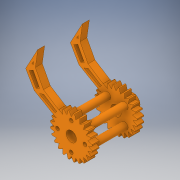
# Autodesk Inventor part: Relic arm front
Saved by Autodesk Inventor 2017 (Build 210142000, 142)
## iProperties
Created: 2018-01-06
Part Number: Relic arm front
Material: Generic
Document SubType Name: Modeling
Designer: Delta
Density: 1 g/cm^3
Appearance: Orange
Author: Delta
Autodesk Inventor part; units mm, degrees
ref_plane "YZ Plane" through (0, 0, 0) normal (1, 0, 0) x (0, 1, 0)
ref_plane "XZ Plane" through (0, 0, 0) normal (0, 1, 0) x (-1, 0, 0)
ref_plane "XY Plane" through (0, 0, 0) normal (0, 0, 1) x (1, 0, 0)
sketch "Sketch1" plane through (0, 0, 0) normal (0, 0, 1) x (1, 0, 0)
  line L0 (0, 0) -> (12.7, 0)
  line L1 (0, 0) -> (12.2673, 3.287)
  line L2 (0, 0) -> (12.7, 0) construction
  line L3 (12.2673, 3.287) -> (19.9534, 1.2275)
  line L4 (12.7, 0) -> (16.4514, 2.1659)
  line L5 (12.7, 0) -> (17.0317, 0) construction
  line L6 (16.4514, 2.1659) -> (12.7, 0)
  line L7 (16.4514, 2.1659) -> (12.2673, 3.287)
  line L8 (0, 0) -> (12.2673, 3.287)
  line L9 (16.4514, 2.1659) -> (12.7, 0)
  line L10 (0, 0) -> (12.7, 0)
  dimension "d0" = 12.7
  dimension "d1" = 12.7
  dimension "d2" = 15
  dimension "d3" = 150
  dimension "d4" = 30
  constraints: 22 end point, 3 horizontal, 2 collinear, 2 equal length, 1 point on line
  measures "d0" distance of L0.start L0.end
  measures "d1" distance of L0.start L1.end
  measures "d2" angle of L2 L1
  measures "d3" angle of L1 L3
  measures "d4" angle of L5 L4
extrude "Extrusion1" add sketch "Sketch1" along normal blind 5.08
sketch "Sketch2" plane through (0, 0, 5.08) normal (0, 0, 1) x (1, 0, 0)
  line L0 (0, 0) -> (12.7, 0) projected
  line L1 (16.4514, 2.1659) -> (12.2673, 3.287) projected
  line L2 (0, 0) -> (12.2673, 3.287)
  line L3 (0, 0) -> (10.9985, 6.35)
  line L4 (0, 0) -> (12.7, 0) construction
  line L5 (12.2673, 3.287) -> (13.7055, 5.7781)
  line L6 (12.2673, 3.287) -> (15.1438, 3.287) construction
  line L7 (13.7055, 5.7781) -> (10.829, 5.7781)
  line L8 (10.9985, 6.35) -> (14.0357, 6.35)
  line L9 (14.0357, 6.35) -> (13.7055, 5.7781)
  line L10 (12.2673, 3.287) -> (15.3303, 6.35)
  line L11 (15.3303, 6.35) -> (14.0357, 6.35)
  line L12 (12.2673, 3.287) -> (15.3303, 6.35)
  line L13 (10.9985, 6.35) -> (15.3303, 6.35)
  dimension "d7" = 12.7
  dimension "d8" = 30
  dimension "d9" = 60
  dimension "d10" = 60
  constraints: 24 end point, 3 horizontal, 2 collinear, 2 equal length, 1 point on line
  measures "d7" distance of L0.start L3.end
  measures "d8" angle of L4 L3
  measures "d9" angle of L6 L5
  measures "d10" angle of L7 L5
extrude "Extrusion2" add sketch "Sketch2" against normal blind 5.08
sketch "Sketch3" plane through (0, 0, 5.08) normal (0, 0, 1) x (1, 0, 0)
  line L0 (0, 0) -> (10.9985, 6.35) projected
  line L1 (0, 0) -> (10.9985, 6.35)
  line L2 (10.9985, 6.35) -> (15.3303, 6.35)
  line L3 (16.4514, 2.1659) -> (12.2673, 3.287) projected
  line L4 (15.3303, 6.35) -> (12.2673, 3.287)
  line L5 (12.7, 0) -> (16.4514, 2.1659) projected
  line L6 (12.2673, 3.287) -> (16.4514, 2.1659)
  line L7 (16.4514, 2.1659) -> (12.7, 0)
  line L8 (12.7, 0) -> (0, 0)
  line L9 (10.9985, 6.35) -> (13.1644, 10.1014)
  line L10 (10.1014, 13.1644) -> (8.9803, 8.9803)
  line L11 (13.1644, 10.1014) -> (8.9803, 8.9803)
  line L12 (6.35, 10.9985) -> (10.1014, 13.1644)
  line L13 (6.35, 10.9985) -> (0, 0)
  line L14 (0, 0) -> (0, 12.7)
  line L15 (0, 12.7) -> (-2.1659, 16.4514)
  line L16 (-6.35, 15.3303) -> (-3.287, 12.2673)
  line L17 (-2.1659, 16.4514) -> (-3.287, 12.2673)
  line L18 (-6.35, 10.9985) -> (-6.35, 15.3303)
  line L19 (-6.35, 10.9985) -> (0, 0)
  line L20 (6.35, 10.9985) -> (6.35, 15.3303)
  line L21 (6.35, 15.3303) -> (3.287, 12.2673)
  line L22 (2.1659, 16.4514) -> (3.287, 12.2673)
  line L23 (0, 12.7) -> (2.1659, 16.4514)
  line L24 (0, 0) -> (-10.9985, -6.35)
  line L25 (-10.9985, -6.35) -> (-13.1644, -10.1014)
  line L26 (-10.1014, -13.1644) -> (-8.9803, -8.9803)
  line L27 (-13.1644, -10.1014) -> (-8.9803, -8.9803)
  line L28 (-6.35, -10.9985) -> (-10.1014, -13.1644)
  line L29 (-6.35, -10.9985) -> (0, 0)
  line L30 (-12.7, 0) -> (0, 0)
  line L31 (-12.7, 0) -> (-16.4514, -2.1659)
  line L32 (-16.4514, -2.1659) -> (-12.2673, -3.287)
  line L33 (-15.3303, -6.35) -> (-12.2673, -3.287)
  line L34 (-10.9985, -6.35) -> (-15.3303, -6.35)
  line L35 (-12.7, 0) -> (-16.4514, 2.1659)
  line L36 (-16.4514, 2.1659) -> (-12.2673, 3.287)
  line L37 (-15.3303, 6.35) -> (-12.2673, 3.287)
  line L38 (-10.9985, 6.35) -> (-15.3303, 6.35)
  line L39 (0, 0) -> (-10.9985, 6.35)
  line L40 (-10.9985, 6.35) -> (-13.1644, 10.1014)
  line L41 (-13.1644, 10.1014) -> (-8.9803, 8.9803)
  line L42 (-10.1014, 13.1644) -> (-8.9803, 8.9803)
  line L43 (-6.35, 10.9985) -> (-10.1014, 13.1644)
  constraints: 82 end point, 28 symmetric about line, 2 collinear, 1 horizontal
extrude "Extrusion3" add sketch "Sketch3" against normal blind 5.08 contours L14 L23 L22 L21 L20 L13 | L19 L18 L16 L17 L15 L14 | L29 L28 L26 L27 L25 L24 | L24 L34 L33 L32 L31 L30
sketch "Sketch4" plane through (0, 0, 5.08) normal (0, 0, 1) x (1, 0, 0)
  line L0 (6.35, 10.9985) -> (0, 0) projected
  line L1 (0, 0) -> (6.35, 10.9985)
  line L2 (6.35, 10.9985) -> (6.35, 15.3303) projected
  line L3 (6.35, 10.9985) -> (6.35, 15.3303)
  line L4 (6.35, 15.3303) -> (3.287, 12.2673)
  line L5 (0, 12.7) -> (2.1659, 16.4514) projected
  line L6 (3.287, 12.2673) -> (2.1659, 16.4514)
  line L7 (2.1659, 16.4514) -> (0, 12.7)
  line L8 (0, 12.7) -> (-2.1659, 16.4514)
  line L9 (-2.1659, 16.4514) -> (0, 12.7) projected
  line L10 (-3.287, 12.2673) -> (-2.1659, 16.4514) projected
  line L11 (-3.287, 12.2673) -> (-6.35, 15.3303)
  line L12 (-6.35, 10.9985) -> (-6.35, 15.3303) projected
  line L13 (-6.35, 15.3303) -> (-6.35, 10.9985)
  line L14 (-6.35, 10.9985) -> (0, 0)
  line L15 (-12.7, 0) -> (0, 0)
  line L16 (-12.7, 0) -> (-16.4514, 2.1659)
  line L17 (-16.4514, 2.1659) -> (-12.2673, 3.287)
  line L18 (-10.9985, 6.35) -> (-15.3303, 6.35)
  line L19 (-12.2673, 3.287) -> (-15.3303, 6.35)
  line L20 (-10.9985, 6.35) -> (-13.1644, 10.1014)
  line L21 (-8.9803, 8.9803) -> (-13.1644, 10.1014)
  line L22 (-8.9803, 8.9803) -> (-10.1014, 13.1644)
  line L23 (-6.35, 10.9985) -> (-10.1014, 13.1644)
  constraints: 37 end point, 8 symmetric about line, 4 collinear, 1 parallel, 1 perpendicular
extrude "Extrusion4" add sketch "Sketch4" against normal blind 5.08 contours L15 L16 L17 L19 L18 L20 L21 L22 L23 L14
sketch "Sketch5" plane through (0, 0, 5.08) normal (0, 0, 1) x (1, 0, 0)
  line L0 (-6.35, -10.9985) -> (0, 0) projected
  line L1 (6.35, 10.9985) -> (0, 0) projected
  line L2 (-6.35, -10.9985) -> (6.35, 10.9985)
  line L3 (6.35, 15.3303) -> (3.287, 12.2673) projected
  line L4 (6.35, 10.9985) -> (6.35, 15.3303)
  line L5 (6.35, 15.3303) -> (3.287, 12.2673)
  line L6 (2.1659, 16.4514) -> (0, 12.7) projected
  line L7 (3.287, 12.2673) -> (2.1659, 16.4514)
  line L8 (2.1659, 16.4514) -> (0, 12.7)
  line L9 (0, 12.7) -> (-2.1659, 16.4514)
  line L10 (-2.1659, 16.4514) -> (-3.287, 12.2673) projected
  line L11 (-2.1659, 16.4514) -> (-3.287, 12.2673)
  line L12 (-3.287, 12.2673) -> (-6.35, 15.3303) projected
  line L13 (-3.287, 12.2673) -> (-6.35, 15.3303)
  line L14 (-6.35, 15.3303) -> (-6.35, 11.0066)
  line L15 (-6.35, 11.0066) -> (-10.0944, 13.1684)
  line L16 (-10.0944, 13.1684) -> (-8.9711, 8.9762)
  line L17 (-8.9711, 8.9762) -> (-13.1633, 10.0995)
  line L18 (-10.9985, 6.35) -> (-13.1644, 10.1014) projected
  line L19 (-13.1633, 10.0995) -> (-10.9985, 6.35)
  line L20 (-15.3303, 6.35) -> (-10.9985, 6.35) projected
  line L21 (-10.9985, 6.35) -> (-15.3303, 6.35)
  line L22 (-16.4514, 2.1659) -> (-12.2673, 3.287) projected
  line L23 (-15.3303, 6.35) -> (-12.2673, 3.287)
  line L24 (-12.2673, 3.287) -> (-16.4514, 2.1659)
  line L25 (-16.4514, 2.1659) -> (-12.7, 0)
  line L26 (-16.4514, -2.1659) -> (-12.7, 0) projected
  line L27 (-12.7, 0) -> (-16.4514, -2.1659)
  line L28 (-16.4514, -2.1659) -> (-12.2673, -3.287) projected
  line L29 (-16.4514, -2.1659) -> (-12.2673, -3.287)
  line L30 (-12.2673, -3.287) -> (-15.3303, -6.35)
  line L31 (-15.3303, -6.35) -> (-10.9985, -6.35) projected
  line L32 (-15.3303, -6.35) -> (-10.9985, -6.35)
  line L33 (-10.9985, -6.35) -> (-13.1644, -10.1014)
  line L34 (-13.1644, -10.1014) -> (-8.9803, -8.9803)
  line L35 (-8.9803, -8.9803) -> (-10.1014, -13.1644)
  line L36 (-10.1014, -13.1644) -> (-6.4778, -11.0723)
  line L37 (-10.1014, -13.1644) -> (-6.35, -10.9985) projected
  line L38 (-6.4778, -11.0723) -> (-6.35, -10.9985)
  line L39 (10.1014, 13.1644) -> (8.9803, 8.9803)
  line L40 (6.35, 10.9985) -> (10.1014, 13.1644)
  line L41 (13.1644, 10.1014) -> (10.9985, 6.35)
  line L42 (8.9803, 8.9803) -> (13.1644, 10.1014)
  line L43 (10.9985, 6.35) -> (15.3303, 6.35)
  line L44 (15.3303, 6.35) -> (12.2673, 3.287)
  line L45 (12.2673, 3.287) -> (16.4514, 2.1659)
  line L46 (16.4514, 2.1659) -> (12.707, 0.0041)
  line L47 (12.707, 0.0041) -> (16.4514, -2.1578)
  line L48 (16.4514, -2.1578) -> (12.2592, -3.2811)
  line L49 (12.2592, -3.2811) -> (15.3281, -6.35)
  line L50 (15.3281, -6.35) -> (10.9985, -6.35)
  line L51 (13.1644, -10.1014) -> (10.9985, -6.35)
  line L52 (10.1014, -13.1644) -> (8.9803, -8.9803)
  line L53 (13.1644, -10.1014) -> (8.9803, -8.9803)
  line L54 (10.1014, -13.1644) -> (6.35, -10.9985)
  line L55 (6.35, -15.3303) -> (6.35, -10.9985)
  line L56 (6.35, -15.3303) -> (3.287, -12.2673)
  line L57 (3.287, -12.2673) -> (2.1659, -16.4514)
  line L58 (2.1659, -16.4514) -> (0, -12.7)
  line L59 (0, -12.7) -> (-2.1659, -16.4514)
  line L60 (-2.1659, -16.4514) -> (-3.287, -12.2673)
  line L61 (-3.287, -12.2673) -> (-6.35, -15.3303)
  line L62 (-6.35, -15.3303) -> (-6.35, -11.1461)
  line L63 (-6.35, -10.9985) -> (-6.35, -11.2315)
  dimension "d17" = 25.4
  constraints: 102 end point, 24 symmetric about line, 10 collinear, 8 point on line, 6 parallel, 2 perpendicular, 1 vertical
  measures "d17" distance of L0.start L1.start
extrude "Extrusion5" add sketch "Sketch5" along normal blind 5.08
sketch "Sketch6" plane through (0, 0, 0) normal (0, 0, -1) x (-1, 0, 0)
  circle A0 centre (0, 0) radius 24.7045
  constraints: 1 centre point, 1 coincident
extrude "Extrusion6" cut sketch "Sketch6" against normal blind 5.08
sketch "Sketch7" plane through (0, 0, 5.08) normal (0, 0, -1) x (-1, 0, 0)
  circle A0 centre (0, 0) radius 3.81
  dimension "d22" = 7.62
  constraints: 1 centre point, 1 coincident
  measures "d22" diameter of A0
extrude "Extrusion7" cut sketch "Sketch7" against normal blind 5.08
sketch "Sketch8" plane through (0, 0, 5.08) normal (0, 0, -1) x (-1, 0, 0)
  circle A0 centre (0, 0) radius 15.6138
  circle A1 centre (0, 0) radius 22.1599
  constraints: 2 centre point, 2 coincident
extrude "Extrusion8" cut sketch "Sketch8" against normal blind 5.08
sketch "Sketch9" plane through (0, 0, 5.08) normal (0, 0, -1) x (-1, 0, 0)
  circle A0 centre (0, 10.16) radius 1.397
  circle A1 centre (-10.16, 0) radius 1.397
  circle A2 centre (0, -10.16) radius 1.397
  circle A3 centre (10.16, 0) radius 1.397
  point P0 (0, 0)
  dimension "d27" = 10.16
  dimension "d28" = 2.794
  dimension "d29" = 10.16
  dimension "d30" = 2.794
  dimension "d31" = 10.16
  dimension "d32" = 10.16
  dimension "d33" = 2.794
  dimension "d34" = 2.794
  constraints: 4 centre point, 4 coincident
  measures "d27" distance of point (0, 0) point (0, 10.16)
  measures "d28" diameter of A0
  measures "d29" distance of point (-10.16, 0) point (0, 0)
  measures "d30" diameter of A1
  measures "d31" distance of point (10.16, 0) point (0, 0)
  measures "d32" distance of point (0, -10.16) point (0, 0)
  measures "d33" diameter of A2
  measures "d34" diameter of A3
extrude "Extrusion9" cut sketch "Sketch9" against normal blind 5.08
sketch "Sketch10" plane through (0, 0, 5.08) normal (0, 0, -1) x (-1, 0, 0)
  circle A0 centre (0, 10.16) radius 1.397 projected
  line L0 (1.397, 10.16) -> (10.16, 1.397)
  circle A1 centre (10.16, 0) radius 1.397 projected
  line L1 (1.397, 10.16) -> (5.7785, 10.16)
  line L2 (10.16, 1.397) -> (10.16, 5.7785)
  line L3 (5.7785, 10.16) -> (24.8285, 43.1556)
  line L4 (5.7785, 10.16) -> (43.8785, 10.16) construction
  line L5 (10.16, 5.7785) -> (27.381, 15.721)
  line L6 (10.16, 5.7785) -> (30.0451, 5.7785) construction
  line L7 (27.381, 15.721) -> (33.731, 26.7196)
  line L8 (33.731, 26.7196) -> (25.1536, 43.7186)
  line L9 (24.8285, 43.1556) -> (33.731, 26.7196)
  line L10 (24.8285, 43.1556) -> (26.5895, 30.8427)
  line L11 (26.5895, 30.8427) -> (20.6258, 19.6212)
  line L12 (20.6258, 19.6212) -> (5.7785, 10.16)
  line L13 (5.7785, 10.16) -> (10.16, 5.7785)
  point P0 (0, 0)
  dimension "d37" = 38.1
  dimension "d38" = 60
  dimension "d39" = 30
  dimension "d40" = 12.7
  dimension "d41" = 150
  constraints: 28 end point, 3 horizontal, 2 equal length, 2 point on circle, 1 horizontal alignment, 1 vertical, 1 other
  measures "d37" distance of L1.end L3.end
  measures "d38" angle of L4 L3
  measures "d39" angle of L6 L5
  measures "d40" distance of L5.end L7.end
  measures "d41" angle of L7 L5
extrude "Extrusion10" add sketch "Sketch10" against normal blind 5.08 contours L12 L11 L10 L9 L7 L5 L13
sketch "Sketch11" plane through (0, 0, 5.08) normal (0, 0, -1) x (-1, 0, 0)
  line L0 (10.8111, 10.6087) -> (11.8256, 9.239)
  line L1 (11.8256, 9.239) -> (23.5441, 15.5294)
  line L2 (23.5441, 15.5294) -> (20.6005, 16.7995)
  line L3 (20.6005, 16.7995) -> (10.8111, 10.6087)
  line L4 (22.6664, 19.3904) -> (26.0333, 17.9377)
  line L5 (26.0333, 17.9377) -> (31.1535, 26.6899)
  line L6 (31.1535, 26.6899) -> (27.5285, 28.8106)
  line L7 (27.5285, 28.8106) -> (22.6664, 19.3904)
  line L8 (28.2363, 28.3965) -> (23.42, 19.0652)
  line L9 (28.0166, 33.9882) -> (29.1302, 31.9137)
  line L10 (29.1302, 31.9137) -> (28.0166, 31.9137)
  line L11 (28.0166, 31.9137) -> (28.0166, 33.9882)
  point P0 (0, 0)
  constraints: 24 end point, 3 perpendicular, 3 point on line, 2 parallel, 1 horizontal
extrude "Extrusion11" cut sketch "Sketch11" against normal blind 5.08 contours L3 L2 L1 L0 | L8 L6 L5 L4 | L9 L10 L11
sketch "Sketch12" plane through (0, 0, 5.08) normal (0, 0, -1) x (-1, 0, 0)
  line L0 (0, 0) -> (-6.4136, 6.4136)
  line L1 (0, 0) -> (9.0702, 0) construction
  circle A0 centre (-6.4136, 6.4136) radius 2.54
  line L2 (0, 0) -> (6.4136, 6.4136)
  line L3 (0, 0) -> (9.0702, 0) construction
  line L4 (0, 0) -> (6.4136, -6.4136)
  line L5 (0, 0) -> (9.0702, 0) construction
  line L6 (0, 0) -> (-6.4136, -6.4136)
  line L7 (0, 0) -> (9.0702, 0) construction
  circle A1 centre (-6.4136, -6.4136) radius 2.54
  circle A2 centre (6.4136, -6.4136) radius 2.54
  circle A3 centre (6.4136, 6.4136) radius 2.54
  dimension "d46" = 135
  dimension "d47" = 5.08
  dimension "d48" = 45
  dimension "d49" = 45
  dimension "d50" = 135
  dimension "d51" = 5.08
  dimension "d52" = 5.08
  dimension "d53" = 5.08
  constraints: 16 end point, 4 centre point, 4 coincident, 4 equal length, 4 horizontal
  measures "d46" angle of L1 L0
  measures "d47" diameter of A0
  measures "d48" angle of L3 L2
  measures "d49" angle of L4 L5
  measures "d50" angle of L6 L7
  measures "d51" diameter of A1
  measures "d52" diameter of A2
  measures "d53" diameter of A3
extrude "Extrusion12" add sketch "Sketch12" along normal blind 27.94
sketch "Sketch13" plane through (6.4136, 6.4136, -22.86) normal (0, 0, -1) x (-1, 0, 0)
  line L0 (19.1136, -6.4136) -> (21.9418, -8.0465) projected
  line L1 (6.4136, -6.4136) -> (19.1136, -6.4136)
  line L2 (18.6809, -3.1266) -> (21.8353, -3.9718) projected
  line L3 (6.4136, -6.4136) -> (18.6809, -3.1266)
  line L4 (18.6809, -3.1266) -> (24.8145, -4.7701)
  line L5 (19.1136, -6.4136) -> (22.865, -4.2477)
  line L6 (19.1136, -6.4136) -> (23.4453, -6.4136) construction
  dimension "d56" = 30
  constraints: 10 end point, 2 horizontal, 1 collinear, 1 equal length, 1 point on line
  measures "d56" angle of L6 L5
extrude "Extrusion13" add sketch "Sketch13" along normal blind 5.08
sketch "Sketch14" plane through (6.4136, 6.4136, -27.94) normal (0, 0, -1) x (-1, 0, 0)
  line L0 (6.4136, -6.4136) -> (19.1136, -6.4136) projected
  line L1 (18.6809, -3.1266) -> (6.4136, -6.4136) projected
  line L2 (6.4136, -6.4136) -> (18.6809, -3.1266)
  line L3 (19.1136, -6.4136) -> (22.865, -4.2477) projected
  line L4 (18.6809, -3.1266) -> (22.865, -4.2477)
  line L5 (22.865, -4.2477) -> (19.1136, -6.4136)
  line L6 (19.1136, -6.4136) -> (6.4136, -6.4136)
  line L7 (18.6809, -9.7006) -> (6.4136, -6.4136)
  line L8 (19.1136, -6.4136) -> (22.865, -8.5795)
  line L9 (18.6809, -9.7006) -> (22.865, -8.5795)
  constraints: 14 end point, 2 collinear, 2 symmetric about line, 1 horizontal
extrude "Extrusion14" add sketch "Sketch14" against normal blind 5.08 contours L0 L8 L9 L7
sketch "Sketch15" plane through (6.4136, 6.4136, -27.94) normal (0, 0, -1) x (-1, 0, 0)
  line L0 (18.6809, -3.1266) -> (6.4136, -6.4136) projected
  line L1 (6.4136, -6.4136) -> (18.6809, -3.1266)
  line L2 (22.865, -4.2477) -> (18.6809, -3.1266) projected
  line L3 (18.6809, -3.1266) -> (22.865, -4.2477)
  line L4 (22.865, -4.2477) -> (19.1136, -6.4136)
  line L5 (19.1136, -6.4136) -> (22.865, -8.5795) projected
  line L6 (19.1136, -6.4136) -> (22.865, -8.5795)
  line L7 (22.865, -8.5795) -> (18.6809, -9.7006)
  line L8 (18.6809, -9.7006) -> (6.4136, -6.4136) projected
  line L9 (18.6809, -9.7006) -> (6.4136, -6.4136)
  line L10 (21.7439, -0.0636) -> (18.6809, -3.1266)
  line L11 (21.7439, -0.0636) -> (17.4121, -0.0636)
  line L12 (17.4121, -0.0636) -> (19.578, 3.6878)
  line L13 (19.578, 3.6878) -> (15.3939, 2.5667)
  line L14 (15.3939, 2.5667) -> (6.4136, -6.4136)
  constraints: 22 end point, 4 collinear, 4 symmetric about line, 1 parallel
extrude "Extrusion15" add sketch "Sketch15" against normal blind 5.08 contours L0 L14 L13 L12 L11 L10
sketch "Sketch16" plane through (6.4136, 6.4136, -27.94) normal (0, 0, -1) x (-1, 0, 0)
  line L0 (15.3939, 2.5667) -> (6.4136, -6.4136) projected
  line L1 (6.4136, -6.4136) -> (15.3939, 2.5667)
  line L2 (19.578, 3.6878) -> (15.3939, 2.5667) projected
  line L3 (15.3939, 2.5667) -> (19.578, 3.6878)
  line L4 (19.578, 3.6878) -> (17.4121, -0.0636) projected
  line L5 (19.578, 3.6878) -> (17.4121, -0.0636)
  line L6 (17.4121, -0.0636) -> (21.7439, -0.0636)
  line L7 (18.6809, -3.1266) -> (21.7439, -0.0636) projected
  line L8 (21.7439, -0.0636) -> (18.6809, -3.1266)
  line L9 (19.1136, -6.4136) -> (22.865, -4.2477) projected
  line L10 (18.6809, -3.1266) -> (22.865, -4.2477)
  line L11 (22.865, -4.2477) -> (19.1136, -6.4136)
  line L12 (19.1136, -6.4136) -> (22.865, -8.5795)
  line L13 (18.6809, -9.7006) -> (20.9901, -12.0098) projected
  line L14 (22.865, -8.5795) -> (18.6809, -9.7006)
  line L15 (6.4136, -6.4136) -> (18.6809, -9.7006) projected
  line L16 (18.6809, -9.7006) -> (6.4136, -6.4136)
  line L17 (16.515, 6.7508) -> (15.3939, 2.5667)
  line L18 (16.515, 6.7508) -> (12.7636, 4.5849)
  line L19 (12.7636, 4.5849) -> (12.7636, 8.9167)
  line L20 (9.7006, 5.8537) -> (12.7636, 8.9167)
  line L21 (6.4136, 6.2864) -> (8.5795, 10.0378)
  line L22 (9.7006, 5.8537) -> (8.5795, 10.0378)
  line L23 (6.4136, 6.2864) -> (4.2477, 10.0378)
  line L24 (4.2477, 10.0378) -> (3.1266, 5.8537)
  line L25 (6.4136, -6.4136) -> (3.1266, 5.8537)
  constraints: 38 end point, 8 symmetric about line, 7 equal length, 1 horizontal, 1 perpendicular
extrude "Extrusion16" add sketch "Sketch16" against normal blind 5.08 contours L0 L25 L24 L23 L21 L22 L20 L19 L18 L17
sketch "Sketch17" plane through (6.4136, 6.4136, -27.94) normal (0, 0, -1) x (-1, 0, 0)
  line L0 (19.578, 3.6878) -> (15.3939, 2.5667) projected
  line L1 (6.4136, -6.4136) -> (15.3939, 2.5667)
  line L2 (15.3939, 2.5667) -> (16.515, 6.7508) projected
  line L3 (15.3939, 2.5667) -> (16.515, 6.7508)
  line L4 (16.515, 6.7508) -> (12.7636, 4.5849) projected
  line L5 (16.515, 6.7508) -> (12.7636, 4.5849)
  line L6 (12.7636, 4.5849) -> (12.7636, 8.9167)
  line L7 (9.7006, 5.8537) -> (8.5795, 10.0378) projected
  line L8 (12.7636, 8.9167) -> (9.7006, 5.8537)
  line L9 (9.7006, 5.8537) -> (8.5795, 10.0378)
  line L10 (4.2477, 10.0378) -> (6.4136, 6.2864) projected
  line L11 (8.5795, 10.0378) -> (6.4136, 6.2864)
  line L12 (6.4136, 6.2864) -> (4.2477, 10.0378)
  line L13 (4.2477, 10.0378) -> (3.1266, 5.8537)
  line L14 (3.1266, 5.8537) -> (6.4136, -6.4136)
  line L15 (6.4136, -6.4136) -> (-5.8537, -3.1266)
  line L16 (-5.8537, -3.1266) -> (-8.9167, -0.0636)
  line L17 (-8.9167, -0.0636) -> (-4.5849, -0.0636)
  line L18 (-4.5849, -0.0636) -> (-6.7508, 3.6878)
  line L19 (-2.5667, 2.5667) -> (-3.6878, 6.7508)
  line L20 (-6.7508, 3.6878) -> (-2.5667, 2.5667)
  line L21 (0.0636, 8.9167) -> (0.0636, 4.5849)
  line L22 (-3.6878, 6.7508) -> (0.0636, 4.5849)
  line L23 (0.0636, 8.9167) -> (3.1266, 5.8537)
  constraints: 38 end point, 8 symmetric about line, 4 collinear, 3 parallel, 1 point on line, 1 vertical
extrude "Extrusion17" add sketch "Sketch17" against normal blind 5.08 contours L15 L16 L17 L18 L20 L19 L22 L21 L23 L14
sketch "Sketch18" plane through (6.4136, 6.4136, -27.94) normal (0, 0, -1) x (-1, 0, 0)
  line L0 (-5.8537, -3.1266) -> (18.6809, -9.7006) projected
  line L1 (-5.8537, -3.1266) -> (18.6809, -9.7006)
  line L2 (22.865, -8.5795) -> (19.1136, -6.4136) projected
  line L3 (18.6809, -9.7006) -> (22.865, -8.5795)
  line L4 (22.865, -8.5795) -> (19.1136, -6.4136)
  line L5 (19.1136, -6.4136) -> (22.865, -4.2477) projected
  line L6 (19.1136, -6.4136) -> (22.865, -4.2477)
  line L7 (22.865, -4.2477) -> (18.6809, -3.1266) projected
  line L8 (22.865, -4.2477) -> (18.6809, -3.1266)
  line L9 (17.4121, -0.0636) -> (21.7439, -0.0636) projected
  line L10 (18.6809, -3.1266) -> (21.7439, -0.0636)
  line L11 (21.7439, -0.0636) -> (17.4121, -0.0636)
  line L12 (17.4121, -0.0636) -> (19.578, 3.6878)
  line L13 (19.578, 3.6878) -> (15.3939, 2.5667) projected
  line L14 (19.578, 3.6878) -> (15.3939, 2.5667)
  line L15 (15.3939, 2.5667) -> (16.515, 6.7508) projected
  line L16 (15.3939, 2.5667) -> (16.515, 6.7508)
  line L17 (16.515, 6.7508) -> (12.8914, 4.6587)
  line L18 (12.7636, 4.5849) -> (12.7636, 8.9167) projected
  line L19 (12.8914, 4.6587) -> (12.7636, 4.5849)
  line L20 (12.7636, 4.5849) -> (12.7636, 8.9167)
  line L21 (12.7636, 8.9167) -> (9.7006, 5.8537) projected
  line L22 (12.7636, 8.9167) -> (9.7006, 5.8537)
  line L23 (9.7006, 5.8537) -> (8.5795, 10.0378)
  line L24 (8.5795, 10.0378) -> (6.4136, 6.2864) projected
  line L25 (6.4136, 6.2864) -> (8.5795, 10.0378)
  line L26 (6.4136, 6.2864) -> (4.2477, 10.0378)
  line L27 (4.2477, 10.0378) -> (3.1266, 5.8537) projected
  line L28 (4.2477, 10.0378) -> (3.1266, 5.8537)
  line L29 (3.1266, 5.8537) -> (0.0636, 8.9167)
  line L30 (0.0636, 4.5849) -> (0.0636, 8.9167) projected
  line L31 (0.0636, 8.9167) -> (0.0636, 4.5849)
  line L32 (-3.6878, 6.7508) -> (0.0636, 4.5849) projected
  line L33 (0.0636, 4.5849) -> (-3.6878, 6.7508)
  line L34 (-2.5667, 2.5667) -> (-3.6878, 6.7508) projected
  line L35 (-3.6878, 6.7508) -> (-2.5667, 2.5667)
  line L36 (-2.5667, 2.5667) -> (-6.7508, 3.6878)
  line L37 (-6.7508, 3.6878) -> (-4.5849, -0.0636)
  line L38 (-5.8537, -3.1266) -> (-8.9167, -0.0636) projected
  line L39 (-4.5849, -0.0636) -> (-8.9167, -0.0636)
  line L40 (-8.9167, -0.0636) -> (-5.8537, -3.1266)
  line L41 (21.7439, -12.7636) -> (17.4121, -12.7636)
  line L42 (18.6809, -9.7006) -> (21.7439, -12.7636)
  line L43 (17.4121, -12.7636) -> (19.578, -16.515)
  line L44 (19.578, -16.515) -> (15.3939, -15.3939)
  line L45 (15.3939, -15.3939) -> (16.515, -19.578)
  line L46 (16.515, -19.578) -> (12.7636, -17.4121)
  line L47 (12.7636, -17.4121) -> (12.7636, -21.7439)
  line L48 (12.7636, -21.7439) -> (9.7006, -18.6809)
  line L49 (9.7006, -18.6809) -> (8.5795, -22.865)
  line L50 (8.5795, -22.865) -> (6.4874, -19.2414)
  line L51 (6.4136, -19.1136) -> (4.2477, -22.865)
  line L52 (6.4874, -19.2414) -> (6.4136, -19.1136)
  line L53 (4.2477, -22.865) -> (3.1266, -18.6809)
  line L54 (3.1266, -18.6809) -> (0.0636, -21.7439)
  line L55 (0.0636, -21.7439) -> (0.0636, -17.4121)
  line L56 (0.0636, -17.4121) -> (-3.6878, -19.578)
  line L57 (-3.6878, -19.578) -> (-2.5667, -15.3939)
  line L58 (-2.5667, -15.3939) -> (-6.7508, -16.515)
  line L59 (-4.5849, -12.7636) -> (-6.7508, -16.515)
  line L60 (-6.7508, -16.515) -> (-4.5849, -12.7636)
  line L61 (-8.9167, -12.7636) -> (-4.5849, -12.7636)
  line L62 (-8.9167, -12.7636) -> (-5.8537, -9.7006)
  line L63 (-5.8537, -9.7006) -> (-10.0378, -8.5795)
  line L64 (-10.0378, -8.5795) -> (-6.2864, -6.4136)
  line L65 (-5.8537, -3.1266) -> (-10.0378, -4.2477)
  line L66 (-6.2864, -6.4136) -> (-10.0378, -4.2477)
  point P0 (6.4136, -6.4136)
  constraints: 106 end point, 24 symmetric about line, 14 collinear, 6 perpendicular, 4 point on line, 3 parallel
extrude "Extrusion18" add sketch "Sketch18" against normal blind 5.08 contours L0 L42 L41 L43 L44 L45 L46 L47 L48 L49 L50 L52 L51 L53 L54 L55 L56 L57 L58 L59 L61 L62 L63 L64 L66 L65
sketch "Sketch19" plane through (6.4136, 6.4136, -27.94) normal (0, 0, -1) x (-1, 0, 0)
  circle A0 centre (6.4136, -6.4136) radius 15.7124
  circle A1 centre (6.4136, -6.4136) radius 23.0018
  constraints: 2 centre point, 2 coincident
extrude "Extrusion19" cut sketch "Sketch19" against normal blind 5.08
sketch "Sketch20" plane through (6.4136, 6.4136, -27.94) normal (0, 0, -1) x (-1, 0, 0)
  circle A0 centre (6.4136, -6.4136) radius 3.81
  dimension "d71" = 7.62
  constraints: 1 centre point, 1 coincident
  measures "d71" diameter of A0
extrude "Extrusion20" cut sketch "Sketch20" against normal blind 5.08
sketch "Sketch21" plane through (6.4136, 6.4136, -27.94) normal (0, 0, -1) x (-1, 0, 0)
  arc A0 (16.267, 5.8252) -> (15.6852, 6.2717) centre (6.4136, -6.4136) ccw projected
  line L0 (33.0031, 24.4291) -> (27.0394, 13.2076) projected
  line L1 (15.9029, 6.1097) -> (27.0394, 13.2076)
  line L2 (27.0394, 13.2076) -> (33.0031, 24.4291)
  line L3 (31.2421, 36.742) -> (33.0031, 24.4291) projected
  line L4 (33.0031, 24.4291) -> (31.2421, 36.742)
  line L5 (33.7946, 9.3074) -> (40.1446, 20.306) projected
  line L6 (31.2421, 36.742) -> (40.1446, 20.306)
  line L7 (40.1446, 20.306) -> (33.7946, 9.3074)
  line L8 (33.7946, 9.3074) -> (17.5445, -0.0636)
  line L9 (17.4121, -0.0636) -> (20.7856, -0.0636) projected
  line L10 (15.9029, 6.1097) -> (12.7011, 0.564)
  line L11 (12.7011, 0.564) -> (17.5445, -0.0636)
  constraints: 16 end point, 3 collinear, 1 parallel, 1 point on circle, 1 point on line
extrude "Extrusion21" add sketch "Sketch21" against normal blind 5.08
sketch "Sketch22" plane through (0, 0, 10.16) normal (0, 0, 1) x (1, 0, 0)
  line L0 (-11.8256, 9.239) -> (-10.8111, 10.6087) projected
  line L1 (-11.8256, 9.239) -> (-23.5788, 15.5159)
  line L2 (-23.5788, 15.5159) -> (-20.6005, 16.7995)
  line L3 (-20.6005, 16.7995) -> (-10.8129, 10.61)
  line L4 (-10.8129, 10.61) -> (-11.8256, 9.239)
  point P0 (0, 0)
  constraints: 8 end point
extrude "Extrusion22" cut sketch "Sketch22" against normal blind 50.8
sketch "Sketch23" plane through (0, 0, 10.16) normal (0, 0, 1) x (1, 0, 0)
  line L0 (-23.42, 19.0652) -> (-26.0333, 17.9377) projected
  line L1 (-26.0333, 17.9377) -> (-23.42, 19.0652)
  line L2 (-31.1535, 26.6899) -> (-28.2363, 28.3965) projected
  line L3 (-23.42, 19.0652) -> (-28.2363, 28.3965)
  line L4 (-28.2363, 28.3965) -> (-31.1535, 26.6899)
  line L5 (-31.1535, 26.6899) -> (-26.0333, 17.9377)
  point P0 (0, 0)
  constraints: 8 end point, 2 collinear, 1 perpendicular
extrude "Extrusion23" cut sketch "Sketch23" against normal blind 50.8
sketch "Sketch24" plane through (0, 0, 10.16) normal (0, 0, 1) x (1, 0, 0)
  line L0 (-28.0166, 31.9137) -> (-29.1302, 31.9137) projected
  line L1 (-28.0166, 31.9137) -> (-28.0166, 33.9731)
  line L2 (-28.0166, 33.9731) -> (-29.1302, 31.9137)
  line L3 (-29.1302, 31.9137) -> (-28.0166, 31.9137)
  point P0 (0, 0)
  constraints: 6 end point, 1 perpendicular, 1 vertical
extrude "Extrusion24" cut sketch "Sketch24" against normal blind 50.8
sketch "Sketch25" plane through (6.4136, 6.4136, -27.94) normal (0, 0, -1) x (-1, 0, 0)
  circle A0 centre (6.4136, -6.4136) radius 7.62
  dimension "d82" = 15.24
  constraints: 1 centre point, 1 coincident
  measures "d82" diameter of A0
extrude "Extrusion25" add sketch "Sketch25" along normal blind 1.27
sketch "Sketch26" plane through (0, 0, -29.21) normal (0, 0, -1) x (-1, 0, 0)
  circle A0 centre (0, 0) radius 5.08
  dimension "d85" = 10.16
  constraints: 1 centre point, 1 coincident
  measures "d85" diameter of A0
extrude "Extrusion26" add sketch "Sketch26" along normal blind 6.35
sketch "Sketch27" plane through (0, 0, -35.56) normal (0, 0, -1) x (-1, 0, 0)
  circle A0 centre (0, 0) radius 3.81
  dimension "d88" = 7.62
  constraints: 1 centre point, 1 coincident
  measures "d88" diameter of A0
extrude "Extrusion27" cut sketch "Sketch27" against normal blind 25.4
body "Solid1"
